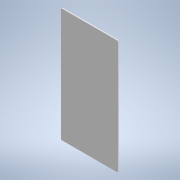
# Autodesk Inventor part: bottom
Saved by Autodesk Inventor 2022 (Build 260153000, 153)
## iProperties
Created: 2022-08-18
Part Number: bottom
Material: Generic
Document SubType Name: Modeling
Designer: HiPeng
Density: 1 g/cm^3
Appearance: Default
Author: HiPeng
Autodesk Inventor part; units mm, degrees
ref_plane "YZ Plane" through (0, 0, 0) normal (1, 0, 0) x (0, 1, 0)
ref_plane "XZ Plane" through (0, 0, 0) normal (0, 1, 0) x (-1, 0, 0)
ref_plane "XY Plane" through (0, 0, 0) normal (0, 0, 1) x (1, 0, 0)
sketch "Sketch1" plane through (0, 0, 0) normal (0, 0, 1) x (1, 0, 0)
  line L0 (299.6071, 149.6071) -> (299.6071, 296.2142)
  arc A0 (299.6071, 296.2142) -> (298.7284, 298.3355) centre (296.6071, 296.2142) ccw
  spline S0 degree 3 poles (298.7284, 298.3355) (298.4498, 298.614) (298.1191, 298.835) (297.3912, 299.1366) (297.001, 299.2142) (296.6071, 299.2142) knots 0 0 0 0 0.5 0.5 1 1 1 1
  line L1 (296.6071, 299.2142) -> (171.4425, 299.2142)
  line L2 (171.4425, 299.2142) -> (153.3929, 299.2142)
  arc A1 (153.3929, 299.2142) -> (150.3929, 296.2142) centre (153.3929, 296.2142) ccw
  line L3 (150.3929, 296.2142) -> (150.3929, 149.6071)
  line L4 (150.3929, 3) -> (150.3929, 149.6071)
  arc A2 (150.3929, 3) -> (153.3929, 0) centre (153.3929, 3) ccw
  line L5 (171.4425, 0) -> (153.3929, 0)
  line L6 (296.6071, 0) -> (171.4425, 0)
  spline S1 degree 3 poles (298.7284, 0.8787) (298.4498, 0.6001) (298.1191, 0.3791) (297.3912, 0.0776) (297.001, 0) (296.6071, 0) knots 0 0 0 0 0.5 0.5 1 1 1 1
  arc A3 (298.7284, 0.8787) -> (299.6071, 3) centre (296.6071, 3) ccw
  line L7 (299.6071, 149.6071) -> (299.6071, 3)
  point P0 (0, 0)
extrude "Extrusion1" add sketch "Sketch1" against normal blind 3
body "Solid1"
